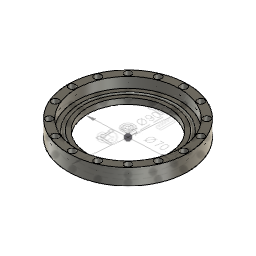
Bottom Base - Ceiling v106 (Autodesk Fusion 360 design; units mm, degrees)
Autodesk Fusion 360 part; units mm, degrees
note: some values were not read from the file. Set by a fixed rule: which sketch regions a step uses; the direction of a hole.
sketch "Sketch2" plane through (0, 0, 0) normal (0, 0, 1) x (1, 0, 0)
  circle A0 centre (0, 0) radius 45 construction
  circle A1 centre (0, 0) radius 52 construction
  circle A2 centre (0, 0) radius 40 construction
  circle A3 centre (0, 0) radius 35 construction
  line L0 (0, 0) -> (0, 52) construction
  line L1 (0, 52) -> (0, 45) construction
  point P0 (0, 48.5)
  point P1 (-18.5601, 44.8082)
  point P2 (-34.2947, 34.2947)
  point P3 (-44.8082, 18.5601)
  point P4 (-48.5, 0)
  point P5 (-44.8082, -18.5601)
  point P6 (-34.2947, -34.2947)
  point P7 (-18.5601, -44.8082)
  point P8 (0, -48.5)
  point P9 (18.5601, -44.8082)
  point P10 (34.2947, -34.2947)
  point P11 (44.8082, -18.5601)
  point P12 (48.5, 0)
  point P13 (44.8082, 18.5601)
  point P14 (34.2947, 34.2947)
  point P15 (18.5601, 44.8082)
  point P16 (0, 40)
  point P17 (28.2843, -28.2843)
  point P18 (36.9552, -15.3073)
  point P19 (40, 0)
  point P20 (36.9552, 15.3073)
  point P21 (28.2843, 28.2843)
  point P22 (15.3073, 36.9552)
  point P23 (-15.3073, 36.9552)
  point P24 (-28.2843, 28.2843)
  point P25 (-36.9552, 15.3073)
  point P26 (-40, 0)
  point P27 (-36.9552, -15.3073)
  point P28 (-28.2843, -28.2843)
  dimension "d80" = 90
  dimension "d81" = 104
  dimension "d82" = 80
  dimension "d83" = 70
  dimension "d85" = 360
  dimension "d87" = 270
  constraint coincident A0.centre A1.centre
  constraint concentric A0 A2
  constraint concentric A2 A3
  constraint coincident A1 L0.end
  constraint vertical L0
  constraint coincident L0 L1.end
  constraint coincident A0 L1.end
  constraint midpoint L1 P0
  constraint coincident A2 P16
  constraint coincident L0 P16
  measures "d80" diameter of A0
  measures "d81" diameter of A1
  measures "d82" diameter of A2
  measures "d83" diameter of A3
sketch "Sketch1" plane through (0, 0, 0) normal (0, 0, 1) x (1, 0, 0) in component "Servo Mount"
  line L0 (0, 0) -> (0, 10.1) construction
  line L1 (-12.35, 10.1) -> (12.35, 10.1)
  line L2 (-12.35, -35.1) -> (-12.35, 10.1)
  line L3 (-12.35, -35.1) -> (12.35, -35.1)
  line L4 (12.35, -35.1) -> (12.35, 10.1)
  line L5 (12.35, -32.74) -> (10.238, -32.74) construction
  line L6 (-12.35, -32.74) -> (-10.238, -32.74) construction
  line L7 (10.238, -32.74) -> (10.238, -8.29) construction
  line L8 (-10.238, -32.74) -> (-10.238, -8.29) construction
  circle A0 centre (-10.238, -8.29) radius 1
  circle A1 centre (10.238, -8.29) radius 1
  circle A2 centre (10.238, -32.74) radius 1
  circle A3 centre (-10.238, -32.74) radius 1
  line L9 (-10.238, -32.74) -> (-10.238, -35.1) construction
  line L10 (10.238, -32.74) -> (10.238, -35.1) construction
  circle A4 centre (0, 0) radius 3.25
  line L11 (0, -35.1) -> (0, -30.3) construction
  line L12 (-12.35, -30.3) -> (12.35, -30.3)
  line L13 (-10.238, -8.29) -> (10.238, -8.29) construction
  line L14 (0, -8.29) -> (0, -11.79) construction
  line L15 (-12.35, -11.79) -> (12.35, -11.79)
  line L16 (-16.35, 14.1) -> (16.35, 14.1)
  line L17 (16.35, -39.1) -> (16.35, 14.1)
  line L18 (-16.35, -39.1) -> (16.35, -39.1)
  line L19 (-16.35, -39.1) -> (-16.35, 14.1)
  circle A5 centre (-10.238, -8.29) radius 2
  circle A6 centre (10.238, -8.29) radius 2
  circle A7 centre (-10.238, -32.74) radius 2
  circle A8 centre (10.238, -32.74) radius 2
  line L20 (0, -35.1) -> (0, -39.1)
  line L21 (0, -11.79) -> (0, -7.79)
  arc A9 (0, -7.79) -> (0, 7.79) centre (0, 0) ccw
  line L22 (0, 7.79) -> (0, 14.1)
  line L23 (0, -35.1) -> (0, -11.79)
  dimension "d1" = 10.1
  dimension "d2" = 24.7
  dimension "d3" = 45.2
  dimension "d5" = 2.112
  dimension "d6" = 2.112
  dimension "d7" = 24.45
  dimension "d8" = 24.45
  dimension "d9" = 2
  dimension "d10" = 2
  dimension "d11" = 2
  dimension "d12" = 2
  dimension "d13" = 2.36
  dimension "d14" = 2.36
  dimension "d15" = 6.5
  dimension "d16" = 4.8
  dimension "d17" = 3.5
  dimension "d18" = 4
  dimension "d31" = 4
  dimension "d32" = 4
  dimension "d33" = 4
  dimension "d34" = 4
  dimension "d69" = 4
  constraint coincident L0.start A4.centre
  constraint vertical L0
  constraint horizontal L1
  constraint midpoint L0.end L1
  constraint vertical L2
  constraint coincident L1.start L2.end
  constraint perpendicular L2 L3
  constraint perpendicular L1 L4
  constraint coincident L4 L5.start
  constraint perpendicular L4 L5
  constraint coincident L2 L6.start
  constraint perpendicular L2 L6
  constraint perpendicular L5 L7
  constraint perpendicular L6 L8
  constraint coincident L8.end A0.centre
  constraint coincident L7.end A1.centre
  constraint coincident L5.end L7.start
  constraint coincident L6.end L8.start
  constraint coincident L3 L9.end
  constraint perpendicular L3 L9
  constraint coincident L3 L10.end
  constraint perpendicular L3 L10
  constraint midpoint L3 L11.start
  constraint perpendicular L3 L11
  constraint coincident L2 L12.start
  constraint coincident L4 L12.end
  constraint perpendicular L4 L12
  constraint midpoint L11.end L12
  constraint midpoint L13 L14.start
  constraint perpendicular L13 L14
  constraint coincident L2 L15.start
  constraint coincident L4 L15.end
  constraint perpendicular L4 L15
  constraint midpoint L14.end L15
  constraint concentric A0 A5
  constraint concentric A1 A6
  constraint concentric A3 A7
  constraint concentric A2 A8
  constraint midpoint L18 L20.end
  constraint perpendicular L15 L21
  constraint coincident L0 A9.end
  constraint midpoint L16 L22.end
  measures "d1" distance of L0.start L0.end
  measures "d2" distance of L1.start L1.end
  measures "d3" distance of L2.start L1.start
  measures "d5" distance of L5.start L5.end
  measures "d6" distance of L6.start L6.end
  measures "d7" distance of L5.end L7.end
  measures "d8" distance of L6.end L8.end
  measures "d9" diameter of A0
  measures "d10" diameter of A1
  measures "d11" diameter of A2
  measures "d12" diameter of A3
  measures "d13" distance of L5.end L10.end
  measures "d14" distance of L6.end L9.end
  measures "d15" diameter of A4
  measures "d16" distance of L11.start L11.end
  measures "d17" distance of L14.start L14.end
  measures "d31" diameter of A5
  measures "d32" diameter of A6
  measures "d33" diameter of A7
  measures "d34" diameter of A8
  measures "d69" distance of L14.end L21.end
extrude "Extrude2" add sketch "Sketch1" along normal blind 16 contours L1 L2 L3 L16 L18 L19 L20 L22 | L1 L3 L4 L16 L17 L18 L20 L22 makes body 1 in component "Servo Mount"
extrude "Extrude4" add sketch "Sketch1" against normal blind 5 separate body contours L1 L2 L3 L16 L18 L19 L20 L22 | L1 L2 L15 L21 A9 L22 | L1 L3 L4 L16 L17 L18 L20 L22 | L1 L4 L15 L21 A9 L22 | L2 L3 L12 L23 | L3 L4 L12 L23 makes body 2 in component "Servo Mount"
extrude "Extrude5" add sketch "Sketch1" against normal blind 2.5 separate body contours A5 | A6 | A7 | A8 makes body 3 at (-8.2405, -32.8397, -1.6667) makes body 4 at (12.2355, -8.3897, -1.6667) makes body 5 at (12.2355, -32.8397, -1.6667) makes body 6 at (-8.2405, -8.3897, -1.6667) in component "Servo Mount"
sketch "Sketch4" plane through (0, -39.1, 0) normal (0, -1, 0) x (1, 0, 0) in component "Servo Mount"
  line L0 (16.35, 0) -> (-16.35, 0)
  line L1 (-16.35, 0) -> (-16.35, -5)
  line L2 (-16.35, -5) -> (16.35, -5)
  line L3 (16.35, -5) -> (16.35, 0)
  line L4 (0, -5) -> (0, -3.75) construction
  line L5 (2.5, -5) -> (-2.5, -5)
  line L6 (-2.5, -5) -> (-2.5, -2.5)
  line L7 (-2.5, -2.5) -> (2.5, -2.5)
  line L8 (2.5, -2.5) -> (2.5, -5)
  line L9 (2.5, -5) -> (-2.5, -2.5) construction
  line L10 (-2.5, -5) -> (2.5, -2.5) construction
  point P0 (0, -3.75)
  dimension "d71" = 1.25
  dimension "d72" = 5
  constraint midpoint L2 L4.start
  constraint perpendicular L2 L4
  constraint perpendicular L5 L6
  constraint parallel L5 L7
  constraint parallel L6 L8
  constraint horizontal L5
  constraint coincident L9 P0
  constraint coincident L10 P0
  constraint coincident P0 L4.end
  constraint collinear L2 L5
  measures "d71" distance of L4.start P0
  measures "d72" distance of L6.end L7.end
sweep "Sweep1" cut profiles "Sketch4" path "Sketch1" along L22 A9 L21 L23 L20 section 1 contours L2 L5 L6 L7 L8 bodies 2 in component "Servo Mount"
sketch "Sketch2 (2)" plane through (0, 0, 0) normal (0, 0, 1) x (1, 0, 0) in component "Servo Mount"
  line L0 (0, 0) -> (0, 10.1) construction
  line L1 (0, 0) -> (-40, 0) construction
  circle A0 centre (-40, 0) radius 5
  circle A1 centre (0, 0) radius 45 construction
  circle A2 centre (0, 0) radius 5 construction
  line L2 (-40.0062, 5) -> (0, 5.05)
  line L3 (-40, -5) -> (0, -5)
  line L4 (0, 0) -> (-30, 0) construction
  circle A3 centre (-30, 0) radius 5 construction
  line L5 (-31.8242, -24.7532) -> (-3.5709, 3.5709)
  circle A4 centre (-28.2843, -28.2843) radius 5
  line L6 (-24.7487, -31.8198) -> (3.5355, -3.5355)
  circle A5 centre (-21.2132, -21.2132) radius 5 construction
  line L7 (0, 0) -> (-21.2132, -21.2132) construction
  line L8 (0, 0) -> (-28.2843, -28.2843) construction
  line L9 (-5, -40.0062) -> (-5.05, 0)
  circle A6 centre (0, -40) radius 5
  line L10 (5, -40) -> (5, 0)
  circle A7 centre (0, -30) radius 5 construction
  line L11 (0, 0) -> (0, -30) construction
  line L12 (0, 0) -> (0, -40) construction
  line L13 (24.7532, -31.8242) -> (-3.5709, -3.5709)
  circle A8 centre (28.2843, -28.2843) radius 5
  line L14 (31.8198, -24.7487) -> (3.5355, 3.5355)
  circle A9 centre (21.2132, -21.2132) radius 5 construction
  line L15 (0, 0) -> (21.2132, -21.2132) construction
  line L16 (0, 0) -> (28.2843, -28.2843) construction
  line L17 (40.0062, -5) -> (0, -5.05)
  circle A10 centre (40, 0) radius 5
  line L18 (40, 5) -> (0, 5)
  circle A11 centre (30, 0) radius 5 construction
  line L19 (0, 0) -> (30, 0) construction
  line L20 (0, 0) -> (40, 0) construction
  line L21 (-16.35, 14.1) -> (16.35, 14.1)
  line L22 (16.35, -39.1) -> (16.35, 14.1)
  line L23 (-16.35, -39.1) -> (-16.35, 14.1)
  line L24 (-16.35, -39.1) -> (16.35, -39.1)
  circle A12 centre (-24.1701, -10) radius 5
  circle A13 centre (24.1619, -10.0198) radius 5
  dimension "d49" = 40
  dimension "d51" = 10
  dimension "d52" = 90
  dimension "d53" = 10
  dimension "d54" = 30
  dimension "d55" = 10
  dimension "d57" = 180
  dimension "d65" = 5
  dimension "d67" = 5
  constraint coincident L0.start L1.start
  constraint perpendicular L0 L1
  constraint coincident L1.end A0.centre
  constraint coincident A0 L2.start
  constraint tangent A0 L2
  constraint midpoint L0 L2.end
  constraint coincident A0 L3.start
  constraint tangent A0 L3
  constraint coincident A2 L3.end
  constraint tangent A2 L3
  constraint perpendicular L0 L4
  constraint coincident L4.end A3.centre
  constraint tangent L3 A12
  constraint tangent L5 A12
  constraint tangent L17 A13
  constraint tangent L14 A13
  measures "d49" distance of L0.start L1.end
  measures "d51" diameter of A0
  measures "d52" diameter of A1
  measures "d53" diameter of A2
  measures "d54" distance of L0.start L4.end
  measures "d55" diameter of A3
  measures "d65" radius of A12
  measures "d67" radius of A13
extrude "Extrude6" add sketch "Sketch2 (2)" along normal blind 6 separate body contours A0 | A0 L2 L3 L23 | L3 L5 L23 A12 | L5 A4 L6 L23 | A4 | L17 A10 L18 L22 | A10 | L14 L17 L22 A13 | L13 A8 L14 L22 | A8 makes body 7 at (26.8352, 1.6601, 0) makes body 8 at (-26.8421, 1.6765, 6) in component "Servo Mount"
sketch "Sketch3" plane through (0, 0, 6) normal (0, 0, 1) x (-1, 0, 0) in component "Servo Mount"
  line L0 (-40, -5) -> (-16.35, -5)
  line L1 (-24.1557, 5.0198) -> (-40.0062, 5)
  arc A0 (-40.0062, 5) -> (-40, -5) centre (-40, 0) ccw
  line L2 (-16.35, -5) -> (-16.35, 23.442)
  line L3 (-16.35, 23.442) -> (-24.7532, 31.8242)
  arc A1 (-24.7532, 31.8242) -> (-31.8198, 24.7487) centre (-28.2843, 28.2843) ccw
  line L4 (-31.8198, 24.7487) -> (-20.6264, 13.5553)
  arc A2 (-24.1557, 5.0198) -> (-20.6264, 13.5553) centre (-24.1619, 10.0198) ccw
  point P0 (40, 0)
  point P1 (30, 0)
  point P2 (28.2843, 28.2843)
  point P3 (21.2132, 21.2132)
  point P4 (-28.2843, 28.2843)
  point P5 (-21.2132, 21.2132)
  point P6 (-40, 0)
  point P7 (-30, 0)
hole "Hole1" at (-28.2843, -28.2843, 6) at (-21.2132, -21.2132, 6) at (-30, 0, 6) at (-40, 0, 6) at (30, 0, 6) at (21.2132, -21.2132, 6) at (40, 0, 6) at (28.2843, -28.2843, 6) direction (0, 0, -1) diameter 2.8 end through all counterbore diameter 6.5 counterbore depth 2.5 bodies 8 7 in component "Servo Mount"
fillet "Fillet3" radius 4 curvature continuous 8 edges at (-16.35, -39.1, 8) (16.35, -39.1, 8) (16.35, 14.1, 8) (-16.35, 14.1, 8) (-16.35, -39.1, -2.5) (16.35, -39.1, -2.5) (-16.35, 14.1, -2.5) (16.35, 14.1, -2.5) on bodies 1 2 in component "Servo Mount"
move_face "OffsetFaces1" offset -0.3 4 faces at (12.35, -20.0333, 5.3333) (-4.1167, 10.1, 10.6667) (-12.35, -20.0333, 5.3333) (-4.1167, -35.1, 10.6667) on bodies 1 in component "Servo Mount"
sketch "Sketch1 (2)" plane through (0, 0, 0) normal (0, 0, 1) x (1, 0, 0) in component "Floor"
  circle A0 centre (0, 0) radius 52
  circle A1 centre (0, 0) radius 45
  circle A2 centre (0, 0) radius 35
  line L0 (16.35, -39.1) -> (16.35, 14.1)
  line L1 (-16.35, -39.1) -> (-16.35, 14.1)
  line L2 (-16.35, -30.9464) -> (-18.35, -30.9464) construction
  line L3 (-18.35, -29.804) -> (-18.35, -41.0887)
  line L4 (18.35, -29.804) -> (18.35, -41.0887)
  line L5 (0, 0) -> (0, 52)
  line L6 (0, 0) -> (0, -48.5) construction
  line L7 (-5, -44.7891) -> (5, -44.7891)
  line L8 (5, -44.7891) -> (5, -52.2109)
  line L9 (5, -52.2109) -> (-5, -52.2109)
  line L10 (-5, -52.2109) -> (-5, -44.7891)
  line L11 (-5, -44.7891) -> (5, -52.2109) construction
  line L12 (5, -44.7891) -> (-5, -52.2109) construction
  point P0 (0, -48.5)
  point P1 (0, -48.5)
  dimension "d89" = 2
  dimension "d90" = 7.4219
  dimension "d91" = 10
  constraint coincident A2 L2.start
  constraint coincident L1 L2.start
  constraint perpendicular L1 L2
  constraint coincident A2 L3.start
  constraint coincident A1 L3.end
  constraint coincident L2.end L3
  constraint vertical L3
  constraint coincident A2 L4.start
  constraint coincident A1 L4.end
  constraint symmetric L3 L4 L5
  constraint coincident A0.centre A1.centre
  constraint coincident P1 P0
  constraint perpendicular L7 L8
  constraint parallel L7 L9
  constraint parallel L8 L10
  constraint horizontal L7
  constraint coincident L11 P1
  constraint coincident L12 P1
  measures "d89" distance of L2.start L2.end
  measures "d90" distance of L7.end L8.end
  measures "d91" distance of L8.end L9.end
extrude "Extrude1" add sketch "Sketch1 (2)" along normal blind 5 separate body contours A1 A2 L3 L5 | A1 A2 L4 L5 makes body 9 in component "Floor"
extrude "Extrude2'" add sketch "Sketch1 (2)" along normal blind 7 separate body contours A0 A1 L5 L7 L8 | A0 A1 L5 L7 L10 | A0 A1 L7 L8 L10 makes body 10 in component "Floor"
hole "Hole1'" at (18.5601, -44.8082, 0) at (34.2947, -34.2947, 0) at (44.8082, -18.5601, 0) at (48.5, 0, 0) at (44.8082, 18.5601, 0) at (34.2947, 34.2947, 0) at (18.5601, 44.8082, 0) at (15.3073, 36.9552, 0) at (28.2843, 28.2843, 0) at (36.9552, 15.3073, 0) at (40, 0, 0) at (36.9552, -15.3073, 0) at (28.2843, -28.2843, 0) at (-18.5601, -44.8082, 0) at (-34.2947, -34.2947, 0) at (-28.2843, -28.2843, 0) at (-36.9552, -15.3073, 0) at (-44.8082, -18.5601, 0) at (-48.5, 0, 0) at (-40, 0, 0) at (-36.9552, 15.3073, 0) at (-44.8082, 18.5601, 0) at (-28.2843, 28.2843, 0) at (-15.3073, 36.9552, 0) at (0, 40, 0) at (0, 48.5, 0) at (-18.5601, 44.8082, 0) at (-34.2947, 34.2947, 0) direction (0, 0, 1) diameter 2.529 end through all counterbore diameter 6.3 counterbore depth 2.5 bodies 10 9 in component "Floor"
thread "Thread1" "ISO Metric profile 3.0 M3x0.5 6H" in component "Floor"
extrude "Extrude3" cut sketch "Sketch1 (2)" along normal blind 5 contours A0 A1 L7 L8 L10 bodies 10 in component "Floor"
sketch "Sketch1 (3)" plane through (0, 0, 0) normal (1, 0, 0) x (0, 1, 0) in component "Ceiling"
  line L0 (35, 0) -> (-35, 0)
  line L1 (52, 0) -> (-52, 0)
  line L2 (45, 0) -> (-45, 0)
  line L3 (40, 0) -> (-40, 0)
  line L4 (-35, 0) -> (-52, 0)
  line L5 (-35, 0) -> (-35, 5)
  line L6 (-35, 5) -> (-45, 5)
  line L7 (-45, 5) -> (-45, 14)
  line L8 (-45, 0) -> (-45, 5) construction
  line L9 (-45, 14) -> (-52, 14)
  line L10 (-52, 14) -> (-52, 0)
  line L11 (-38.6025, 5) -> (-41.3975, 5) construction
  line L12 (-40, 5) -> (-40, 4.45) construction
  arc A0 (-41.3975, 5) -> (-38.6025, 5) centre (-40, 6.5005) ccw
  dimension "d106" = 5
  dimension "d107" = 9
  dimension "d108" = 2.795
  dimension "d109" = 0.55
  constraint coincident L0.end L4.start
  constraint coincident L1.end L4.end
  constraint perpendicular L4 L5
  constraint perpendicular L5 L6
  constraint perpendicular L6 L7
  constraint coincident L2.end L8.start
  constraint perpendicular L6 L8
  constraint perpendicular L7 L9
  constraint perpendicular L4 L10
  constraint perpendicular L8 L11
  constraint midpoint L6 L12.start
  constraint perpendicular L6 L12
  constraint midpoint L11 L12.start
  constraint coincident L12.end A0
  measures "d106" distance of L0.end L5.end
  measures "d107" distance of L6.end L7.end
  measures "d108" distance of L11.start L11.end
  measures "d109" distance of L12.start L12.end
revolve "Revolve1" add sketch "Sketch1 (3)" angle 360 about axis through (0, 0, 1.75) along (0, 0, 1) separate body contours L1 L2 L3 L4 L5 L6 L7 L9 L10 A0 makes body 11 in component "Ceiling"
sketch "Sketch2 (3)" plane through (0, 0, 14) normal (0, 0, 1) x (-1, 0, 0) in component "Ceiling"
  circle A0 centre (0, 0) radius 52
  circle A1 centre (0, 0) radius 45
  point P0 (0, -48.5)
  point P1 (-18.5601, -44.8082)
  point P2 (-34.2947, -34.2947)
  point P3 (-44.8082, -18.5601)
  point P4 (-48.5, 0)
  point P5 (-44.8082, 18.5601)
  point P6 (-34.2947, 34.2947)
  point P7 (-18.5601, 44.8082)
  point P8 (0, 48.5)
  point P9 (18.5601, 44.8082)
  point P10 (34.2947, 34.2947)
  point P11 (44.8082, 18.5601)
  point P12 (48.5, 0)
  point P13 (44.8082, -18.5601)
  point P14 (34.2947, -34.2947)
  point P15 (18.5601, -44.8082)
hole "Hole1''" at (-34.2947, -34.2947, 14) at (-44.8082, -18.5601, 14) at (-48.5, 0, 14) at (-44.8082, 18.5601, 14) at (-34.2947, 34.2947, 14) at (-18.5601, 44.8082, 14) at (0, 48.5, 14) at (18.5601, 44.8082, 14) at (34.2947, 34.2947, 14) at (44.8082, 18.5601, 14) at (48.5, 0, 14) at (44.8082, -18.5601, 14) at (34.2947, -34.2947, 14) at (18.5601, -44.8082, 14) at (0, -48.5, 14) at (-18.5601, -44.8082, 14) direction (0, 0, -1) diameter 2.8 end through all counterbore diameter 6.1 counterbore depth 5 bodies 11 in component "Ceiling"
move_face "OffsetFaces1'" offset -0.1 1 faces at (-2.2431, -44.9441, 8) on bodies 11 in component "Ceiling"
component "Servo Mount" placed x (1, 0, 0) y (0, 1, 0) z (0, 0, 1) at (0, 0, 0)
component "Floor" placed x (1, 0, 0) y (0, 1, 0) z (0, 0, 1) at (0, 0, 0)
component "Ceiling" placed x (1, 0, 0) y (0, 1, 0) z (0, 0, 1) at (0, 0, 0)
component "Turntable" placed x (1, 0, 0) y (0, 1, 0) z (0, 0, 1) at (0, 0, 0)
component "Bearing Guide" placed x (1, 0, 0) y (0, 1, 0) z (0, 0, 1) at (0, 0, 0)
equation "shout = shin + 14 mm"
equation "shin = prim + 10 mm"
equation "prim = 80 mm"
equation "inner = prim - 10 mm"
equation "sinkh = 2.5 mm" comment "Depth of a countersink"
equation "sinkw = 6.5 mm" comment "Diameter of a countersink"
equation "d47 = -sinkh"
equation "d49 = prim / 2"
equation "buffer = prim - inner" comment "Diameter of things like supports"
equation "d51 = buffer"
equation "d52 = shin"
equation "d55 = buffer"
equation "d63 = sinkh"
equation "d64 = sinkw"
equation "d65 = buffer / 2"
equation "d67 = buffer / 2"
equation "d80 = shin"
equation "d81 = shout"
equation "d82 = prim"
equation "d83 = inner"
equation "ceildrop = 9 mm" comment "The space between ceiling top and bearing support rim"
equation "trackh = 0.55 mm"
equation "trackw = 2.795 mm"
equation "d107 = ceildrop"
equation "d108 = trackw"
equation "d109 = trackh"
